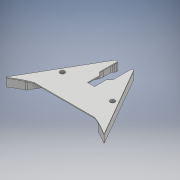
# Autodesk Inventor part: Delta motor covers wire cutout
Saved by Autodesk Inventor 2018 (Build 220112000, 112)
## iProperties
Created: 2018-02-11
Part Number: Delta motor covers wire cutout
Material: Generic
Document SubType Name: Modeling
Designer: elect
Density: 1 g/cm^3
Appearance: Default
Author: elect
Autodesk Inventor part; units mm, degrees
ref_plane "YZ Plane" through (0, 0, 0) normal (1, 0, 0) x (0, 1, 0)
ref_plane "XZ Plane" through (0, 0, 0) normal (0, 1, 0) x (-1, 0, 0)
ref_plane "XY Plane" through (0, 0, 0) normal (0, 0, 1) x (1, 0, 0)
sketch "Sketch1" plane through (0, 0, 0) normal (0, 0, 1) x (1, 0, 0)
  arc A0 (-65.4012, 176.2816) -> (-106.8297, 154.7254) centre (-0.0106, 0.0202) ccw
  line L0 (106.8196, 154.7177) -> (18.9207, 306.9805)
  line L1 (-0.077, 176.3062) -> (65.2471, 176.3308)
  line L2 (-0.077, 176.3062) -> (-65.4012, 176.2816)
  line L3 (-0.077, 233.6594) -> (7.6346, 233.6594)
  line L4 (7.6346, 233.6594) -> (7.6346, 259.6594)
  line L5 (-0.077, 233.6594) -> (-7.577, 233.6594)
  line L6 (-7.577, 233.6594) -> (-7.577, 259.7218)
  line L7 (-7.577, 259.7218) -> (-14.6481, 266.7929)
  line L8 (7.6346, 259.6594) -> (14.7057, 266.7305)
  line L9 (-14.6481, 266.7929) -> (-14.6481, 307.0429)
  line L10 (14.7057, 266.7305) -> (14.7057, 306.9805)
  line L11 (-106.8297, 154.7254) -> (-18.8626, 307.0429)
  arc A1 (106.8196, 154.7177) -> (65.2471, 176.3308) centre (-0.0106, 0.0202) ccw
  arc A2 (-106.8297, 154.7254) -> (-106.8378, 154.7198) centre (-0.0106, 0.0202) ccw
  line L12 (-14.6481, 309.7929) -> (-14.6481, 309.7305)
  line L13 (-14.6481, 307.0429) -> (-18.8626, 307.0429)
  line L14 (14.7057, 307.0429) -> (14.7057, 306.9805)
  line L15 (14.7057, 306.9805) -> (18.9207, 306.9805)
  point P0 (0, 0)
  dimension "d39" = 175.8943
  dimension "d40" = 4.2146
  dimension "d41" = 40.25
  dimension "d73" = 4.215
  dimension "d75" = 40.25
  constraints: 32 end point, 8 point on circle, 3 centre point, 3 perpendicular, 2 horizontal, 2 point on line, 2 vertical
  measures "d39" distance of L11.start L11.end
  measures "d40" distance of L9.end L11.end
  measures "d41" distance of L7.end L9.end
  measures "d73" distance of L10.end L0.end
  measures "d75" distance of L8.end L10.end
extrude "Extrusion1" add sketch "Sketch1" along normal blind 2
sketch "Sketch2" plane through (0, 0, 0) normal (0, 0, -1) x (-1, 0, 0)
  line L0 (0, 0) -> (188, 0) construction
  line L1 (106.8086, 154.7124) -> (18.8616, 307.041)
  line L2 (-106.8086, 154.7124) -> (-18.8616, 307.041)
  line L3 (-18.8616, 307.041) -> (-14.6466, 307.041)
  line L4 (18.8616, 307.041) -> (14.6466, 307.041)
  line L5 (-77.6518, 171.2139) -> (-48.1129, 222.3768)
  line L6 (-77.6518, 171.2139) -> (-18.8616, 273.0414)
  line L7 (14.6466, 280.342) -> (18.8616, 273.0414)
  arc A0 (106.8086, 154.7124) -> (77.6518, 171.2139) centre (0, 0) ccw
  arc A1 (-77.6518, 171.2139) -> (-106.8086, 154.7124) centre (0, 0) ccw
  line L8 (-18.8616, 297.041) -> (-18.8616, 273.0414)
  line L9 (18.8616, 297.041) -> (18.8616, 273.0414)
  line L10 (-14.6466, 307.041) -> (-14.6466, 302.041)
  line L11 (-14.6466, 302.041) -> (-18.8616, 297.041)
  line L12 (14.6466, 307.041) -> (14.6466, 302.041)
  line L13 (18.8616, 297.041) -> (14.6466, 302.041)
  line L14 (-18.8616, 273.0414) -> (-14.6466, 280.342)
  line L15 (18.8616, 273.0414) -> (77.6518, 171.2139)
  dimension "d45" = 4.215
  dimension "d66" = 126.0103
  dimension "d68" = 175.894
  dimension "d69" = 126.0103
  dimension "d74" = 4.215
  dimension "d121" = 5
  constraints: 32 end point, 4 point on circle, 3 horizontal, 2 centre point, 1 coincident, 1 point on line
  measures "d45" distance of L2.end L3.end
  measures "d66" distance of L5.start L14.end
  measures "d68" distance of L1.start L1.end
  measures "d69" distance of L7.start L15.end
  measures "d74" distance of L1.end L4.end
  measures "d121" distance of L3.end L10.end
extrude "Extrusion2" add sketch "Sketch2" along normal blind 16
fillet "Fillet1" radius 5 2 edges at (18.8616, 307.041, -8) (18.9207, 306.9805, 1)
fillet "Fillet2" radius 5 2 edges at (-18.8616, 307.041, -8) (-18.8626, 307.0429, 1)
fillet "Fillet3" radius 2 1 edges at (14.6466, 307.041, -8)
fillet "Fillet4" radius 2 2 edges at (-14.6466, 307.041, -8) (-14.6481, 307.0429, 1)
fillet "Fillet5" radius 5 1 edges at (-77.6518, 171.2139, -8)
fillet "Fillet6" radius 5 1 edges at (77.6518, 171.2139, -8)
sketch "Sketch3" plane through (0, 0, 2) normal (0, 0, 1) x (1, 0, 0)
  circle A0 centre (0, 0) radius 188
  line L0 (0, 0) -> (-106.8086, 154.7124)
  line L1 (0, 0) -> (188, 0) construction
  line L2 (0, 0) -> (106.8086, 154.7124)
  line L3 (106.8086, 154.7124) -> (18.8616, 307.041)
  line L4 (106.8086, 154.7124) -> (282.7026, 154.7124) construction
  line L5 (18.8616, 307.041) -> (10.2014, 302.041)
  line L6 (10.2014, 302.041) -> (54.1749, 225.8767)
  line L7 (-106.8086, 154.7124) -> (-18.6825, 307.041)
  line L8 (-18.6825, 307.041) -> (-10.0267, 302.0334)
  line L9 (-10.0267, 302.0334) -> (-54.0673, 225.9079)
  dimension "d88" = 376
  dimension "d89" = 124.62
  dimension "d90" = 175.894
  dimension "d91" = 120
  dimension "d92" = 10
  dimension "d93" = 87.947
  dimension "d94" = 90
  dimension "d95" = 10
  dimension "d96" = 87.947
  dimension "d97" = 175.9836
  constraints: 20 end point, 4 perpendicular, 2 equal length, 2 horizontal, 2 point on circle, 1 centre point, 1 coincident
  measures "d88" diameter of A0
  measures "d89" angle of L1 L0
  measures "d90" distance of L2.end L3.end
  measures "d91" angle of L4 L3
  measures "d92" distance of L3.end L5.end
  measures "d93" distance of L5.end L6.end
  measures "d94" angle of L6 L5
  measures "d95" distance of L7.end L8.end
  measures "d96" distance of L8.end L9.end
  measures "d97" distance of L0.end L7.end
hole "Hole1" at (-54.0673, 225.9079, 2) at (54.1749, 225.8767, 2) direction (0, 0, -1) diameter 5 depth 18 tip angle 118 counterbore diameter 10 counterbore depth 13
fillet "Fillet13" radius 20 1 edges at (18.8616, 273.0414, -8)
fillet "Fillet14" radius 20 1 edges at (-18.8616, 273.0414, -8)
fillet "Fillet15" radius 5 1 edges at (-14.6466, 302.041, -8)
fillet "Fillet16" radius 5 1 edges at (14.6466, 302.041, -8)
fillet "Fillet17" radius 5 1 edges at (18.8616, 297.041, -8)
fillet "Fillet18" radius 5 1 edges at (-18.8616, 297.041, -8)
fillet "Fillet19" radius 1 7 edges at (49.198, 220.4973, 0) (77.6774, 171.531, 0) (19.5431, 273.224, 0) (18.8616, 286.8076, 0) (18.5581, 296.9302, 0) (16.7541, 299.541, 0) (15.0958, 301.7961, 0)
fillet "Fillet20" radius 1 7 edges at (-49.198, 220.4973, 0) (-19.5431, 273.224, 0) (-18.8616, 286.8076, 0) (-18.5581, 296.9302, 0) (-16.7541, 299.541, 0) (-14.9711, 302.0955, 0) (-77.6408, 171.5674, 0)
fillet "Fillet21" radius 0.5 2 edges at (-106.8086, 154.7124, -8) (-106.8297, 154.7254, 1)
fillet "Fillet22" radius 0.5 2 edges at (106.8086, 154.7124, -8) (106.8196, 154.7177, 1)
body "Solid1"
